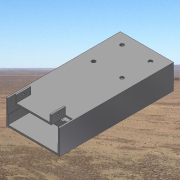
# Autodesk Inventor part: 2p1h37
Saved by Autodesk Inventor 2014 SP1 (Build 180222100, 222)
## iProperties
Company: HERA Project
Created: 2013-12-03
Part Number: 2p1h37
Material: Steel, Galvanized
Document SubType Name: Modeling
Designer: David DeBoer
Mass: 1294.21 g
Surface Area: 1098.03 cm^2
Volume: 164.867 cm^3
Density: 7.85 g/cm^3
Description: end holder 37 degree
Appearance: Galvanized
Author: David DeBoer
Autodesk Inventor part; units mm, degrees
ref_plane "YZ Plane" through (0, 0, 0) normal (1, 0, 0) x (0, 1, 0)
ref_plane "XZ Plane" through (0, 0, 0) normal (0, 1, 0) x (-1, 0, 0)
ref_plane "XY Plane" through (0, 0, 0) normal (0, 0, 1) x (1, 0, 0)
sketch "Sketch1" plane through (0, 0, 0) normal (0, 0, 1) x (1, 0, 0)
  line L0 (0, 0) -> (88.9, 0)
  line L1 (88.9, 0) -> (88.9, 38.1)
  line L2 (88.9, 38.1) -> (0, 38.1)
  line L3 (0, 38.1) -> (0, 0)
  line L4 (-3.048, 41.148) -> (91.948, 41.148)
  line L5 (91.948, 41.148) -> (91.948, -3.048)
  line L6 (91.948, -3.048) -> (-3.048, -3.048)
  line L7 (-3.048, -3.048) -> (-3.048, 41.148)
  dimension "d0" = 88.9
  dimension "d1" = 38.1
  dimension "d2" = 3.048
  constraints: 16 end point, 4 parallel, 2 perpendicular, 1 horizontal, 3 other
  measures "d0" distance of L0.start L0.end
  measures "d1" distance of L2.end L0.start
  measures "d2" distance between parallel lines of L4 L2
extrude "Extrusion1" add sketch "Sketch1" along normal blind 203.2
sketch "Sketch3" plane through (-3.048, 41.148, 0) normal (0, 1, 0) x (1, 0, 0)
  line L0 (0, 0) -> (0, -203.2) projected
  line L1 (94.996, -203.2) -> (0, -203.2) projected
  line L2 (15.24, -203.2) -> (17.78, -203.2)
  line L3 (17.78, -203.2) -> (17.78, -177.8)
  line L4 (17.78, -177.8) -> (15.24, -177.8)
  line L5 (15.24, -177.8) -> (15.24, -203.2)
  line L6 (47.498, -203.2) -> (47.498, -149.4712) construction
  line L7 (79.756, -203.2) -> (77.216, -203.2)
  line L8 (77.216, -203.2) -> (77.216, -177.8)
  line L9 (77.216, -177.8) -> (79.756, -177.8)
  line L10 (79.756, -177.8) -> (79.756, -203.2)
  point P0 (3.048, 0)
  dimension "d10" = 2.54
  dimension "d11" = 25.4
  dimension "d12" = 15.24
  constraints: 18 end point, 4 symmetric about line, 3 parallel, 1 horizontal, 1 midpoint, 1 perpendicular, 1 point on line
  measures "d10" distance of L2.start L2.end
  measures "d11" distance of L2.end L3.end
  measures "d12" distance between parallel lines of L0 L5
extrude "Extrusion3" add sketch "Sketch3" along normal blind 12.7
sketch "Sketch4" plane through (-3.048, 41.148, 0) normal (0, 1, 0) x (1, 0, 0)
  line L0 (77.216, -203.2) -> (17.78, -203.2) projected
  line L1 (15.24, -203.2) -> (0, -203.2) projected
  line L2 (15.24, -177.8) -> (2.54, -177.8)
  line L3 (2.54, -177.8) -> (2.54, -203.2)
  line L4 (2.54, -203.2) -> (15.24, -203.2)
  line L5 (15.24, -203.2) -> (15.24, -177.8)
  line L6 (47.498, -203.2) -> (47.498, -154.3799) construction
  line L7 (79.756, -203.2) -> (79.756, -177.8)
  line L8 (79.756, -177.8) -> (92.456, -177.8)
  line L9 (92.456, -177.8) -> (92.456, -203.2)
  line L10 (92.456, -203.2) -> (79.756, -203.2)
  line L11 (79.756, -203.2) -> (79.756, -177.8)
  point P0 (3.048, 0)
  dimension "d15" = 12.7
  constraints: 20 end point, 4 symmetric about line, 3 parallel, 1 horizontal, 1 midpoint, 1 perpendicular, 1 point on line
  measures "d15" distance of L4.end L3.end
extrude "Extrusion4" cut sketch "Sketch4" against normal blind 25.4
sketch "Sketch5" plane through (0, 0, 0) normal (0, 1, 0) x (1, 0, 0)
  line L0 (0, 0) -> (0, -203.2) projected
  line L1 (88.9, -203.2) -> (0, -203.2) projected
  line L2 (31.75, -161.29) -> (57.15, -161.29)
  line L3 (57.15, -161.29) -> (57.15, -158.75)
  line L4 (57.15, -158.75) -> (31.75, -158.75)
  line L5 (31.75, -158.75) -> (31.75, -161.29)
  dimension "d18" = 25.4
  dimension "d19" = 31.75
  dimension "d20" = 44.45
  dimension "d21" = 2.54
  constraints: 8 end point, 2 parallel, 1 horizontal, 1 perpendicular
  measures "d18" distance of L4.end L3.end
  measures "d19" distance between parallel lines of L5 L0
  measures "d20" distance between parallel lines of L1 L4
  measures "d21" distance of L2.end L3.end
extrude "Extrusion5" add sketch "Sketch5" along normal blind 12.7
sketch "Sketch6" plane through (0, 0, 0) normal (0, 1, 0) x (1, 0, 0)
  line L0 (31.75, -158.75) -> (57.15, -158.75)
  line L1 (57.15, -158.75) -> (57.15, -146.05)
  line L2 (57.15, -146.05) -> (31.75, -146.05)
  line L3 (31.75, -146.05) -> (31.75, -158.75)
  dimension "d24" = 25.4
  dimension "d25" = 12.7
  constraints: 8 end point, 2 parallel, 1 horizontal, 1 perpendicular
  measures "d24" distance of L2.end L1.end
  measures "d25" distance of L1.end L0.end
extrude "Extrusion6" cut sketch "Sketch6" against normal blind 12.7
sketch "Sketch7" plane through (12.192, 38.1, 203.2) normal (-1, 0, 0) x (0, 0, 1)
  line L0 (-25.4, 15.748) -> (0, 15.748) projected
  circle A0 centre (-12.7, 10.668) radius 0.6717
  point P0 (-203.2, -38.1)
  dimension "d28" = 5.08
  constraints: 1 centre point
  measures "d28" distance from line of A0.centre L0
hole "Hole1" at (12.192, 48.768, 190.5) direction (1, 0, 0) diameter 3.302 end through all thread size "8-32 UNC" class "2B" standard "ANSI Unified Screw Threads"
sketch "Sketch8" plane through (-3.048, 41.148, 0) normal (0, 1, 0) x (1, 0, 0)
  line L0 (0, 0) -> (94.996, 0) projected
  circle A0 centre (22.098, -19.05) radius 3.565
  line L1 (3.048, 0) -> (3.048, -177.8) projected
  circle A1 centre (72.898, -19.05) radius 3.565
  circle A2 centre (22.098, -69.85) radius 3.565
  circle A3 centre (72.898, -69.85) radius 3.565
  dimension "d36" = 19.05
  dimension "d38" = 19.05
  dimension "d41" = 50.8
  dimension "d44" = 50.8
  constraints: 4 centre point, 1 horizontal, 1 vertical, 6 other
  measures "d36" distance from line of L0 A0.centre
  measures "d38" distance from line of L1 A0.centre
  measures "d41" distance of A0.centre A1.centre
  measures "d44" distance of A0.centre A2.centre
hole "Hole2" at (19.05, 41.148, 19.05) at (69.85, 41.148, 19.05) at (69.85, 41.148, 69.85) at (19.05, 41.148, 69.85) direction (0, -1, 0) diameter 6.7564 depth 25.4 tip angle 118 clearance for "Flat Head Machine Screw (82)" size "1/4" standard "Ansi Unified Screw Threads"
body "Solid1"
